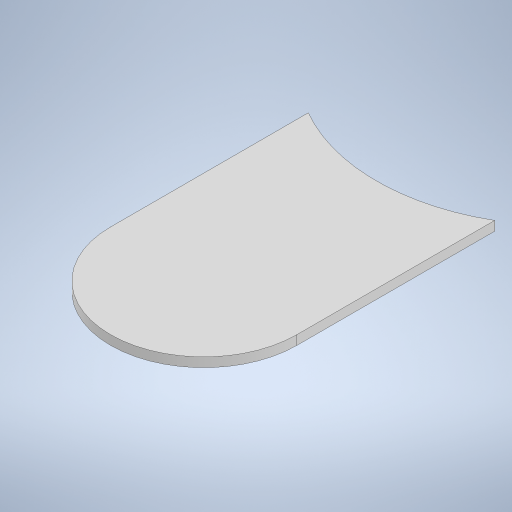
# Autodesk Inventor part: Tapa general
Saved by Autodesk Inventor 2024 (Build 280153000, 153)
## iProperties
Created: 2024-04-29
Part Number: Tapa general
Material: Generic
Document SubType Name: Modeling
Designer: samue
Density: 1 g/cm^3
Appearance: Default
Author: samue
Autodesk Inventor part; units mm, degrees
ref_plane "YZ Plane" through (0, 0, 0) normal (1, 0, 0) x (0, 1, 0)
ref_plane "XZ Plane" through (0, 0, 0) normal (0, 1, 0) x (-1, 0, 0)
ref_plane "XY Plane" through (0, 0, 0) normal (0, 0, 1) x (1, 0, 0)
sketch "Sketch1" plane through (0, 0, 0) normal (0, 1, 0) x (-1, 0, 0)
  arc A0 (30, 0) -> (-30, 0) centre (0, 0) ccw
  line L0 (30, 0) -> (30, -63.6642)
  line L1 (-30, 0) -> (-30, -63.6642)
  arc A1 (30, -63.6642) -> (-30, -63.6642) centre (0, -115.6257) ccw
  dimension "d0" = 60
  dimension "d1" = 60
  constraints: 4 end point, 4 point on circle, 2 centre point, 2 tangent, 2 vertical, 1 coincident
  measures "d0" diameter of A0
  measures "d1" radius of A1
extrude "Extrusion1" add sketch "Sketch1" along normal blind 3
body "Solid1"
